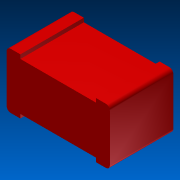
# Autodesk Inventor part: SPDT Toggle Switch Base
Saved by Autodesk Inventor 2011 SP1 (Build 150282100, 282)
## iProperties
Created: 2011-11-07
Part Number: SPDT Toggle Switch Base
Document SubType Name: Modeling
Designer: sdarley
Density: 1 g/cm^3
Author: sdarley
Autodesk Inventor part; units mm, degrees
ref_plane "YZ Plane" through (0, 0, 0) normal (1, 0, 0) x (0, 1, 0)
ref_plane "XZ Plane" through (0, 0, 0) normal (0, 1, 0) x (-1, 0, 0)
ref_plane "XY Plane" through (0, 0, 0) normal (0, 0, 1) x (1, 0, 0)
sketch "Sketch1" plane through (0, 0, 0) normal (0, 0, 1) x (1, 0, 0)
  line L0 (-6.5, 4) -> (6.5, 4)
  line L1 (6.5, 4) -> (6.5, -4)
  line L2 (6.5, -4) -> (-6.5, -4)
  line L3 (-6.5, -4) -> (-6.5, 4)
  point P0 (0, 0)
  point P1 (-6.5, 0)
  point P2 (0, -4)
  dimension "d0" = 8
  dimension "d1" = 13
  constraints: 8 end point, 2 midpoint, 2 parallel, 1 horizontal, 1 horizontal alignment, 1 perpendicular, 1 vertical alignment
  measures "d0" distance between parallel lines of L0 L2
  measures "d1" distance between parallel lines of L1 L3
extrude "Extrusion1" add sketch "Sketch1" along normal blind 7
sketch "Sketch2" plane through (-6.5, 4, 0) normal (0, 1, 0) x (1, 0, 0)
  line L0 (0, -7) -> (13, -7) projected
  line L1 (0, 0) -> (13, 0) projected
  line L2 (11.275, -7) -> (1.725, -7)
  line L3 (1.725, -7) -> (1.725, -6.5)
  line L4 (1.725, -6.5) -> (11.275, -6.5)
  line L5 (11.275, -6.5) -> (11.275, -7)
  line L6 (11.275, 0) -> (1.725, 0)
  line L7 (1.725, 0) -> (1.725, -0.5)
  line L8 (1.725, -0.5) -> (11.275, -0.5)
  line L9 (11.275, -0.5) -> (11.275, 0)
  line L10 (1.725, -0.05) -> (11.275, -0.05) projected
  line L11 (1.725, -0.3) -> (1.725, -0.05) projected
  line L12 (0.5, -0.3) -> (1.725, -0.3) projected
  line L13 (0, -0.8) -> (0.5, -0.3) projected
  line L14 (0, -6.2) -> (0, -0.8) projected
  line L15 (0.5, -6.7) -> (0, -6.2) projected
  line L16 (1.725, -6.7) -> (0.5, -6.7) projected
  line L17 (1.725, -6.7) -> (1.725, -6.75) projected
  line L18 (11.275, -6.75) -> (1.725, -6.75) projected
  line L19 (11.275, -6.7) -> (11.275, -6.75) projected
  line L20 (12.5, -6.7) -> (11.275, -6.7) projected
  line L21 (13, -6.2) -> (12.5, -6.7) projected
  line L22 (13, -0.8) -> (13, -6.2) projected
  line L23 (12.5, -0.3) -> (13, -0.8) projected
  line L24 (11.275, -0.3) -> (12.5, -0.3) projected
  line L25 (11.275, -0.3) -> (11.275, -0.05) projected
  point P0 (6.5, 0)
  point P1 (6.5, -7)
  point P2 (6.5, -7)
  point P3 (6.5, -0.5)
  point P4 (6.5, 0)
  dimension "d4" = 0.5
  dimension "d5" = 0.5
  dimension "d6" = 9.55
  dimension "d7" = 9.55
  constraints: 16 end point, 4 midpoint, 4 parallel, 2 horizontal, 2 perpendicular, 2 point on line, 1 coincident, 1 vertical alignment
  measures "d4" distance of L2.end L3.end
  measures "d5" distance of L7.end L6.end
  measures "d6" distance between parallel lines of L3 L5
  measures "d7" distance between parallel lines of L7 L9
extrude "Extrusion2" cut sketch "Sketch2" against normal through all contours L3 L18 L5 L0 | L3 L4 L5 L18 | L7 L10 L9 L8 | L7 L1 L9 L10
fillet "Fillet1" radius 0.5 4 edges at (6.5, 0, 7) (6.5, 0, 0) (-6.5, 0, 0) (-6.5, 0, 7)
equation "\"d7\" = d6"
body "Solid1"
